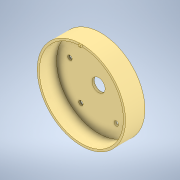
# Autodesk Inventor part: Wheel_1
Saved by Autodesk Inventor 2020.1 (Build 241239000, 239)
## iProperties
Created: 2020-01-18
Part Number: Wheel_1
Material: Generic
Document SubType Name: Modeling
Designer: Ali
Density: 1 g/cm^3
Appearance: Default
Author: Ali
Autodesk Inventor part; units mm, degrees
ref_plane "YZ Plane" through (0, 0, 0) normal (1, 0, 0) x (0, 1, 0)
ref_plane "XZ Plane" through (0, 0, 0) normal (0, 1, 0) x (-1, 0, 0)
ref_plane "XY Plane" through (0, 0, 0) normal (0, 0, 1) x (1, 0, 0)
sketch "Sketch1" plane through (0, 0, 0) normal (0, 0, 1) x (1, 0, 0)
  circle A0 centre (0, 0) radius 130.175
  dimension "d0" = 260.35
  constraints: 1 centre point, 1 coincident
  measures "d0" diameter of A0
extrude "Extrusion1" add sketch "Sketch1" along normal blind 6.35
sketch "Sketch2" plane through (0, 0, 6.35) normal (0, 0, 1) x (1, 0, 0)
  circle A0 centre (0, 0) radius 130.175 projected
  circle A1 centre (0, 0) radius 123.825
  dimension "d3" = 6.35
  constraints: 1 centre point
  measures "d3" radial gap between concentric circles of A0 A1
extrude "Extrusion2" add sketch "Sketch2" along normal blind 50.8
sketch "Sketch4" plane through (0, 0, 6.35) normal (0, 0, 1) x (1, 0, 0)
  point P0 (0, 0)
  point P1 (0, 0)
  constraints: 1 coincident
hole "Hole1" at (0, 0, 6.35) direction (0, 0, -1) diameter 38.608 end through all
sketch "Sketch5" plane through (0, 0, 6.35) normal (0, 0, 1) x (1, 0, 0)
  point P0 (0, 0)
  point P1 (0, 88.9)
  dimension "d13" = 88.9
  measures "d13" distance of point (0, 0) point (0, 88.9)
hole "Hole2" at (0, 88.9, 6.35) direction (0, 0, -1) diameter 13.208 end through all
pattern_circular "Circular Pattern1" count 5 over 360 about axis through (0, 0, -366.2495) along (0, 0, 1) of "Hole2"
sketch "Sketch7" plane through (-0.7894, 85.7534, 57.15) normal (0, 0, 1) x (1, 0, 0)
  line L0 (-3.175, 44.45) -> (3.175, 44.45)
  line L1 (3.175, 44.45) -> (3.175, 38.1)
  line L2 (3.175, 38.1) -> (-3.175, 38.1)
  line L3 (-3.175, 38.1) -> (-3.175, 44.45)
  point P0 (0, 0)
  dimension "d35" = 6.35
  dimension "d36" = 6.35
  dimension "d33" = 3.175
  dimension "d34" = 44.45
  constraints: 8 end point, 2 parallel, 1 horizontal, 1 perpendicular
  measures "d35" distance of L1.end L2.end
  measures "d36" distance of L0.end L1.end
  measures "d33" distance from line of point (0, 0) L3
  measures "d34" distance from line of point (0, 0) L0
extrude "Extrusion4" add sketch "Sketch7" along normal blind 6.35
fillet "Fillet1" radius 2.54 4 edges at (-0.7894, 130.2034, 63.5) (2.3856, 127.0284, 63.5) (-0.7894, 123.8534, 63.5) (-3.9644, 127.0284, 63.5)
equation "\"d0\" = W_innerDiameter + W_wallThickness"
equation "\"d1\" = W_wallThickness"
equation "\"d3\" = W_wallThickness"
equation "\"d4\" = W_innerDepth"
equation "\"d6\" = W_innerGearHoleDiameter"
equation "\"d13\" = OG_distanceFromCenter"
equation "\"d14\" = W_outerGearHoleDiameter"
equation "\"d33\" = 0.5 * d35"
equation "\"d34\" = 0.35 * d40"
equation "\"d39\" = d41"
equation "\"W_wallThickness\" = 6.35"
equation "\"W_innerDepth\" = 50.8"
equation "\"W_innerGearHoleDiameter\" = 38.608"
equation "\"W_outerGearHoleDiameter\" = 13.208"
equation "\"OG_distanceFromCenter\" = 88.9"
equation "\"W_innerDiameter\" = 254"
equation "\"Wheel_Related_W_\" = 0"
equation "\"W_holesClearance\" = 0.254"
equation "\"TempSpotReserved7\" = 0"
equation "\"TempSpotReserved8\" = 0"
equation "\"TempSpotReserved9\" = 0"
equation "\"TempSpotReserved10\" = 0"
equation "\"TempSpotReserved11\" = 0"
equation "\"TempSpotReserved12\" = 0"
equation "\"TempSpotReserved13\" = 0"
equation "\"TempSpotReserved14\" = 0"
equation "\"TempSpotReserved15\" = 0"
equation "\"TempSpotReserved16\" = 0"
equation "\"TempSpotReserved17\" = 0"
equation "\"TempSpotReserved18\" = 0"
equation "\"TempSpotReserved19\" = 0"
equation "\"TempSpotReserved20\" = 0"
equation "\"Inner_Gear_Related_IG_\" = 0"
equation "\"IG_shaftDiameter\" = 25.4"
equation "\"IG_gearDiameter\" = 127"
equation "\"IG_shaftLength\" = 76.2"
equation "\"IG_gearThickness\" = 6.35"
equation "\"TempSpotReserved25\" = 0"
equation "\"TempSpotReserved26\" = 0"
equation "\"TempSpotReserved27\" = 0"
equation "\"TempSpotReserved28\" = 0"
equation "\"TempSpotReserved29\" = 0"
equation "\"TempSpotReserved30\" = 0"
equation "\"TempSpotReserved31\" = 0"
equation "\"TempSpotReserved32\" = 0"
equation "\"TempSpotReserved33\" = 0"
equation "\"TempSpotReserved34\" = 0"
equation "\"TempSpotReserved35\" = 0"
equation "\"TempSpotReserved36\" = 0"
equation "\"TempSpotReserved37\" = 0"
equation "\"TempSpotReserved38\" = 0"
equation "\"TempSpotReserved39\" = 0"
equation "\"TempSpotReserved40\" = 0"
equation "\"Outer_Gear_Related_OG_\" = 0"
equation "\"OG_shaftDiameter\" = 12.7"
equation "\"OG_gearDiameter\" = 50.8"
equation "\"OG_shaftLength\" = 57.15"
equation "\"OG_gearThickness\" = 6.35"
equation "\"TempSpotReserved47\" = 0"
equation "\"TempSpotReserved48\" = 0"
equation "\"TempSpotReserved49\" = 0"
equation "\"TempSpotReserved50\" = 0"
equation "\"TempSpotReserved51\" = 0"
equation "\"TempSpotReserved52\" = 0"
equation "\"TempSpotReserved53\" = 0"
equation "\"TempSpotReserved54\" = 0"
equation "\"TempSpotReserved55\" = 0"
equation "\"TempSpotReserved56\" = 0"
equation "\"TempSpotReserved57\" = 0"
equation "\"TempSpotReserved58\" = 0"
equation "\"TempSpotReserved59\" = 0"
equation "\"TempSpotReserved60\" = 0"
equation "\"Leg_Extensions_Related_LE_\" = 0"
equation "\"LE_baseDiameter\" = 19.05"
equation "\"LE_maxLength\" = 93.92488"
equation "\"LE_thickness\" = 19.05"
equation "\"IG_ratioToOuterGear\" = 2.5"
equation "\"B_bearingThickness\" = 6.35"
equation "\"TempSpotReserved43\" = 0"
equation "\"TempSpotReserved45\" = 0"
equation "\"Thisisatest\" = 25.4"
equation "\"TempSpotReserved46\" = 0"
equation "\"TempSpotReserved44\" = 0"
equation "\"LE_offsetAboveOuterGear\" = 0"
equation "\"Bearing_Related_B_\" = 0"
equation "\"TempSpotReserved42\" = 0"
equation "\"d41\" = 6.35"
equation "\"d40\" = 127"
body "Solid1"
